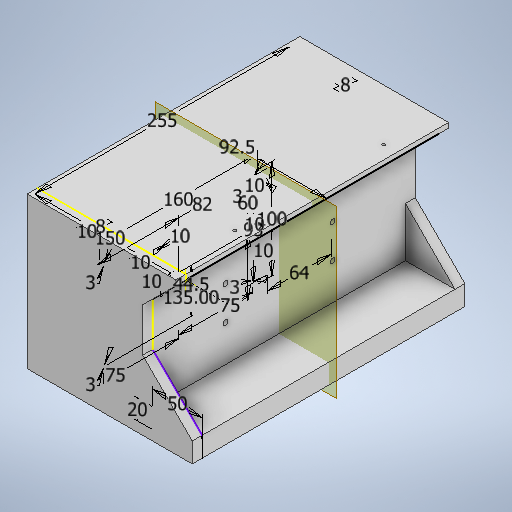
# Autodesk Inventor part: EboxCase
Saved by Autodesk Inventor 2025.1 (Build 291241000, 241)
## iProperties
Created: 2025-02-21
Part Number: EboxCase
Material: Generic
Document SubType Name: Modeling
Designer: m_kni
Density: 1 g/cm^3
Appearance: Default
Author: m_kni
Autodesk Inventor part; units mm, degrees
ref_plane "YZ Plane" through (0, 0, 0) normal (1, 0, 0) x (0, 1, 0)
ref_plane "XZ Plane" through (0, 0, 0) normal (0, 1, 0) x (-1, 0, 0)
ref_plane "XY Plane" through (0, 0, 0) normal (0, 0, 1) x (1, 0, 0)
sketch "Sketch1" plane through (0, 0, 0) normal (0, 1, 0) x (-1, 0, 0)
  line L0 (-75, -127.5) -> (75, -127.5)
  line L1 (75, -127.5) -> (75, 127.5)
  line L2 (75, 127.5) -> (-75, 127.5)
  line L3 (-75, 127.5) -> (-75, -127.5)
  line L4 (-75, -127.5) -> (75, 127.5) construction
  line L5 (75, -127.5) -> (-75, 127.5) construction
  line L6 (-75, 0) -> (-36.5, 0)
  line L7 (-41.5, -127.5) -> (-31.5, -127.5)
  line L8 (-31.5, -127.5) -> (-31.5, 127.5)
  line L9 (-31.5, 127.5) -> (-41.5, 127.5)
  line L10 (-41.5, 127.5) -> (-41.5, -127.5)
  line L11 (-41.5, -127.5) -> (-31.5, 127.5) construction
  line L12 (-31.5, -127.5) -> (-41.5, 127.5) construction
  line L13 (12.5, -127.5) -> (22.5, -127.5)
  line L14 (22.5, -127.5) -> (22.5, 127.5)
  line L15 (22.5, 127.5) -> (12.5, 127.5)
  line L16 (12.5, 127.5) -> (12.5, -127.5)
  line L17 (12.5, -127.5) -> (22.5, 127.5) construction
  line L18 (22.5, -127.5) -> (12.5, 127.5) construction
  line L19 (75, 127.5) -> (22.1863, 127.5)
  line L20 (22.1863, 127.5) -> (22.1863, 119.5)
  line L21 (22.1863, 119.5) -> (75, 119.5)
  line L22 (75, 119.5) -> (75, 127.5)
  line L23 (75, -127.5) -> (22.1863, -127.5)
  line L24 (22.1863, -127.5) -> (22.1863, -119.5)
  line L25 (22.1863, -119.5) -> (75, -119.5)
  line L26 (75, -119.5) -> (75, -127.5)
  line L27 (12.8137, -119.5) -> (-31.5, -119.5)
  line L28 (-31.5, -119.5) -> (-31.5, -127.5)
  line L29 (-31.5, -127.5) -> (12.8137, -127.5)
  line L30 (12.8137, -127.5) -> (12.8137, -119.5)
  line L31 (22.1863, 119.5) -> (-31.5, 119.5)
  line L32 (-31.5, 119.5) -> (-31.5, 127.5)
  line L33 (-31.5, 127.5) -> (22.1863, 127.5)
  line L34 (22.1863, 127.5) -> (22.1863, 119.5)
  point P0 (0, 0)
  point P1 (17.5, 0)
  point P2 (22.5, -119.5)
  point P3 (22.5, 119.5)
  point P4 (-31.5, -119.5)
  point P5 (12.5, 119.5)
  point P6 (12.5, -119.5)
  dimension "d0" = 150
  dimension "d1" = 255
  dimension "d3" = 10
  dimension "d4" = 92.5
  dimension "d5" = 10
  dimension "d6" = 8
  dimension "d7" = 8
  constraints: 70 end point, 14 parallel, 8 horizontal, 7 midpoint, 7 perpendicular, 5 point on line
  measures "d0" distance of L2.end L1.end
  measures "d1" distance of L1.end L0.end
  measures "d3" distance of L9.end L8.end
  measures "d4" distance from line of point (17.5, 0) L3
  measures "d5" distance of L15.end L14.end
  measures "d6" distance of L20.end L19.end
  measures "d7" distance of L23.end L24.end
extrude "Extrusion1" add sketch "Sketch1" along normal blind 5
extrude "Extrusion2" add sketch "Sketch1" against normal blind 147.5 contours L10 L2 L8 L0 | L8 L27 L16 L0 | L16 L27 L30 L0 | L30 L27 L16 L31 L21 L14 L25 L24 L0 | L8 L2 L16 L31 | L24 L25 L14 L0 | L16 L2 L20 L31 | L14 L25 L1 L0 | L20 L2 L14 L21 | L14 L2 L1 L21
sketch "Sketch2" plane through (41.5, -147.5, 127.5) normal (1, 0, 0) x (0, 0, -1)
  line L0 (255, 152.5) -> (255, 0) projected
  line L1 (0, 0) -> (0, 152.5) projected
  line L2 (255, 0) -> (0, 0)
  line L3 (0, 0) -> (0, 147.5)
  line L4 (0, 147.5) -> (255, 147.5)
  line L5 (255, 147.5) -> (255, 0)
  line L6 (255, 73.75) -> (0, 73.75)
  line L7 (127.5, 73.75) -> (127.5, 36.343)
  line L8 (73.5, 73.75) -> (73.5, 56.75)
  line L9 (181.5, 73.75) -> (181.5, 56.75)
  line L10 (73.5, 73.75) -> (73.5, 90.75)
  line L11 (181.5, 73.75) -> (181.5, 90.75)
  circle A0 centre (181.5, 56.75) radius 2.5
  circle A1 centre (181.5, 90.75) radius 2.5
  circle A2 centre (73.5, 90.75) radius 2.5
  circle A3 centre (73.5, 56.75) radius 2.5
  point P0 (127.5, 147.5)
  point P1 (127.5, 55.0465)
  point P2 (73.5, 60.2872)
  dimension "d12" = 54
  dimension "d13" = 17
  dimension "d14" = 5
  dimension "d15" = 5
  dimension "d16" = 5
  dimension "d17" = 5
  constraints: 20 end point, 4 centre point, 4 coincident, 4 midpoint, 4 symmetric about line, 2 parallel, 2 point on line, 2 vertical, 1 horizontal, 1 perpendicular
  measures "d12" horizontal distance of L8.start point (127.5, 55.047)
  measures "d13" distance of L8.start L8.end
  measures "d14" diameter of A0
  measures "d15" diameter of A1
  measures "d16" diameter of A2
  measures "d17" diameter of A3
extrude "Extrusion3" cut sketch "Sketch2" against normal blind 147.5 contours A0 | A1 | A2 | A3
sketch "Sketch3" plane through (-22.5, -147.5, -119.5) normal (-1, 0, 0) x (0, 0, 1)
  point P0 (119.5, 147.5)
sketch "Sketch4" plane through (-22.5, -147.5, -119.5) normal (-1, 0, 0) x (0, 0, 1)
  circle A0 centre (173.5, 90.75) radius 2.5 projected
  circle A1 centre (173.5, 56.75) radius 2.5 projected
  circle A2 centre (65.5, 90.75) radius 2.5 projected
  circle A3 centre (65.5, 56.75) radius 2.5 projected
  circle A4 centre (173.5, 90.75) radius 5
  circle A5 centre (173.5, 56.75) radius 5
  circle A6 centre (65.5, 90.75) radius 5
  circle A7 centre (65.5, 56.75) radius 5
  line L0 (237, 10) -> (77, 10)
  line L1 (77, 10) -> (77, 110)
  line L2 (77, 110) -> (237, 110)
  line L3 (237, 110) -> (237, 10)
  line L4 (237, 10) -> (77, 110) construction
  line L5 (77, 10) -> (237, 110) construction
  line L6 (239, 147.5) -> (239, 0) projected
  line L7 (239, 0) -> (0, 0) projected
  line L8 (3, 106.5) -> (67, 106.5)
  line L9 (67, 106.5) -> (67, 13.5)
  line L10 (67, 13.5) -> (3, 13.5)
  line L11 (3, 13.5) -> (3, 106.5)
  line L12 (3, 106.5) -> (67, 13.5) construction
  line L13 (67, 106.5) -> (3, 13.5) construction
  line L14 (157, 60) -> (147.6244, 60)
  line L15 (147.6244, 60) -> (147.6244, 51.0165)
  line L16 (157, 60) -> (157, 51.0165)
  circle A8 centre (232, 15.5) radius 1.5
  circle A9 centre (232, 104.5) radius 1.5
  circle A10 centre (82, 15.5) radius 1.5
  circle A11 centre (82, 104.5) radius 1.5
  point P0 (119.5, 147.5)
  point P1 (35, 60)
  point P2 (157, 10)
  point P3 (232, 10)
  point P4 (82, 10)
  dimension "d20" = 10
  dimension "d21" = 10
  dimension "d22" = 10
  dimension "d23" = 10
  dimension "d24" = 160
  dimension "d25" = 100
  dimension "d26" = 82
  dimension "d27" = 60
  dimension "d28" = 64
  dimension "d29" = 93
  dimension "d30" = 10
  dimension "d31" = 75
  dimension "d32" = 75
  dimension "d33" = 44.5
  dimension "d34" = 3
  dimension "d35" = 3
  dimension "d36" = 3
  dimension "d37" = 3
  constraints: 30 end point, 8 centre point, 8 coincident, 5 midpoint, 4 parallel, 3 horizontal, 3 perpendicular, 3 symmetric about line, 2 point on line, 1 vertical
  measures "d20" diameter of A4
  measures "d21" diameter of A5
  measures "d22" diameter of A6
  measures "d23" diameter of A7
  measures "d24" distance of L1.end L2.end
  measures "d25" distance of L0.end L1.end
  measures "d26" distance from line of L14.start L6
  measures "d27" distance from line of L14.start L7
  measures "d28" distance of L9.end L10.end
  measures "d29" distance of L8.end L9.end
  measures "d30" distance between parallel lines of L9 L1
  measures "d31" distance of point (232, 10) point (157, 10)
  measures "d32" distance of point (82, 10) point (157, 10)
  measures "d33" vertical distance of point (232, 15.5) L14.start
  measures "d34" diameter of A8
  measures "d35" diameter of A9
  measures "d36" diameter of A10
  measures "d37" diameter of A11
extrude "Extrusion4" cut sketch "Sketch4" against normal blind 10 contours A8 | A9 | A10 | A11
sketch "Sketch5" plane through (-75, 5, 127.5) normal (0, 0, 1) x (1, 0, 0)
  line L0 (150, -5) -> (118.233, -36.767)
  line L1 (150, -5) -> (194.9254, -5) construction
  line L2 (118.233, -36.767) -> (116.5, -38.5)
  line L3 (116.5, -5) -> (116.5, -152.5) projected
  line L4 (116.5, -152.5) -> (116.5, -132.5)
  line L5 (116.5, -132.5) -> (166.5, -132.5)
  line L6 (116.5, -152.5) -> (166.5, -152.5)
  line L7 (166.5, -152.5) -> (166.5, -132.5)
  line L8 (116.5, -5) -> (150, -5) projected
  line L9 (150, -5) -> (150, 0) projected
  line L10 (0, 0) -> (150, 0) projected
  line L11 (0, -152.5) -> (0, 0) projected
  line L12 (116.5, -152.5) -> (0, -152.5) projected
  line L13 (116.5, -5) -> (116.5, -152.5) projected
  line L14 (166.5, -132.5) -> (116.5, -82.5)
  point P0 (75, -5)
  dimension "d40" = 135
  dimension "d41" = 20
  dimension "d42" = 50
  constraints: 16 end point, 4 point on line, 3 horizontal, 1 equal length, 1 perpendicular
  measures "d40" angle of L0 L1
  measures "d41" distance of L3.end L4.end
  measures "d42" distance of L4.end L5.end
extrude "Extrusion5" add sketch "Sketch5" along normal blind 10
ref_plane "Work Plane1" through (-22.5, 0, 0) normal (0, 0, -1) x (-1, 0, 0)
mirror "Mirror1" about plane through (-22.5, 0, 0) normal (0, 0, -1) of "Extrusion5"
extrude "Extrusion6" add sketch "Sketch5" against normal up to surface (255 mm away) contours L5 L7 L6 L3
sketch "Sketch6" plane through (0, 0, 0) normal (0, -1, 0) x (1, 0, 0)
  line L0 (75, 127.5) -> (75, -127.5) projected
  line L1 (41.5, 127.5) -> (75, 127.5) projected
  circle A0 centre (61.5, -85.5) radius 1.5
  circle A1 centre (61.5, 64.5) radius 1.5
  point P0 (0, 0)
  dimension "d47" = 13.5
  dimension "d48" = 63
  dimension "d49" = 150
  dimension "d50" = 3
  dimension "d51" = 3
  constraints: 2 centre point, 2 coincident
  measures "d47" distance from line of point (61.5, 64.5) L0
  measures "d48" distance from line of point (61.5, 64.5) L1
  measures "d49" distance of point (61.5, -85.5) point (61.5, 64.5)
  measures "d50" diameter of A0
  measures "d51" diameter of A1
extrude "Extrusion7" cut sketch "Sketch6" against normal blind 10
ref_plane "Work Plane2" through (-22.5, 0, 0) normal (0, 0, -1) x (-1, 0, 0)
body "Solid1"
